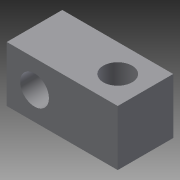
# Autodesk Inventor part: roller_joint
Saved by Autodesk Inventor 2015 (Build 190159000, 159)
## iProperties
Created: 2017-12-05
Part Number: roller_joint
Material: Generic
Document SubType Name: Modeling
Designer: Anshul
Density: 1 g/cm^3
Appearance: Default
Author: Anshul
Autodesk Inventor part; units mm, degrees
ref_plane "YZ Plane" through (0, 0, 0) normal (1, 0, 0) x (0, 1, 0)
ref_plane "XZ Plane" through (0, 0, 0) normal (0, 1, 0) x (-1, 0, 0)
ref_plane "XY Plane" through (0, 0, 0) normal (0, 0, 1) x (1, 0, 0)
sketch "Sketch1" plane through (0, 0, 0) normal (0, 1, 0) x (-1, 0, 0)
  line L0 (0, 0) -> (0, -10)
  line L1 (0, -10) -> (20, -10)
  line L2 (20, -10) -> (20, 0)
  line L3 (20, 0) -> (0, 0)
  line L4 (0, -5) -> (5, -5)
  circle A0 centre (5, -5) radius 2.6
  dimension "d0" = 10
  dimension "d1" = 20
  dimension "d2" = 5
  dimension "d3" = 5.2
  constraints: 10 end point, 3 perpendicular, 1 centre point, 1 coincident, 1 horizontal, 1 midpoint, 1 vertical
  measures "d0" distance of L0.start L0.end
  measures "d1" distance of L0.end L1.end
  measures "d2" distance of L4.start L4.end
  measures "d3" diameter of A0
extrude "Extrusion1" add sketch "Sketch1" along normal blind 10
sketch "Sketch2" plane through (-20, 0, 0) normal (0, 0, 1) x (1, 0, 0)
  line L0 (0, 10) -> (0, 0)
  line L1 (0, 0) -> (0, 10) projected
  line L2 (0, 5) -> (5, 5)
  circle A0 centre (5, 5) radius 2.6
  point P0 (20, 0)
  dimension "d6" = 5
  dimension "d7" = 5.2
  constraints: 4 end point, 1 centre point, 1 coincident, 1 collinear, 1 horizontal, 1 midpoint
  measures "d6" distance of L2.start L2.end
  measures "d7" diameter of A0
extrude "Extrusion2" cut sketch "Sketch2" against normal blind 11
body "Solid1"
